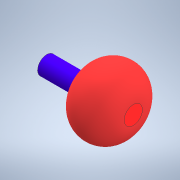
# Autodesk Inventor part: knob
Saved by Autodesk Inventor 2021 (Build 250183000, 183)
## iProperties
Created: 2021-07-29
Part Number: knob
Material: Generic
Document SubType Name: Modeling
Designer: Shammy Haider
Density: 1 g/cm^3
Appearance: Default
Author: Shammy Haider
Autodesk Inventor part; units mm, degrees
ref_plane "YZ Plane" through (0, 0, 0) normal (1, 0, 0) x (0, 1, 0)
ref_plane "XZ Plane" through (0, 0, 0) normal (0, 1, 0) x (-1, 0, 0)
ref_plane "XY Plane" through (0, 0, 0) normal (0, 0, 1) x (1, 0, 0)
sketch "Sketch1" plane through (0, 0, 0) normal (0, 0, 1) x (1, 0, 0)
  line L0 (0, 2.38) -> (10, 2.38)
  arc A0 (22.6233, 2.38) -> (10, 2.38) centre (16.3116, 2.38) ccw
  line L1 (22.6233, 2.38) -> (22.6233, 0)
  line L2 (22.6233, 0) -> (0, 0)
  line L3 (0, 0) -> (0, 2.38)
  dimension "d0" = 2.38
  dimension "d1" = 10
  constraints: 8 end point, 3 perpendicular, 2 point on circle, 2 point on line, 1 centre point, 1 horizontal, 1 tangent
  measures "d0" distance between parallel lines of L0 L2
  measures "d1" distance of L0.start L0.end
revolve "Revolution1" add sketch "Sketch1" angle 360 about axis through (22.6233, 0, 0) along (-1, 0, 0)
body "Solid1"
